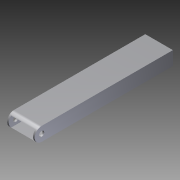
# Autodesk Inventor part: apendage arm
Saved by Autodesk Inventor 2012 (Build 160160000, 160)
## iProperties
Created: 2013-09-04
Part Number: apendage arm
Material: Default
Document SubType Name: Modeling
Designer: Bryce
Density: 1 g/cm^3
Author: Bryce
Autodesk Inventor part; units mm, degrees
ref_plane "YZ Plane" through (0, 0, 0) normal (1, 0, 0) x (0, 1, 0)
ref_plane "XZ Plane" through (0, 0, 0) normal (0, 1, 0) x (-1, 0, 0)
ref_plane "XY Plane" through (0, 0, 0) normal (0, 0, 1) x (1, 0, 0)
sketch "Sketch1" plane through (0, 0, 0) normal (0, 0, 1) x (1, 0, 0)
  line L0 (0, 0) -> (50.8, 0)
  line L1 (50.8, 0) -> (50.8, 25.4)
  line L2 (50.8, 25.4) -> (0, 25.4)
  line L3 (0, 25.4) -> (0, 0)
  line L4 (3.175, 3.175) -> (47.625, 3.175)
  line L5 (47.625, 3.175) -> (47.625, 22.225)
  line L6 (47.625, 22.225) -> (3.175, 22.225)
  line L7 (3.175, 22.225) -> (3.175, 3.175)
  dimension "d0" = 25.4
  dimension "d1" = 50.8
  dimension "d2" = 3.175
  dimension "d3" = 3.175
  dimension "d4" = 3.175
  dimension "d5" = 3.175
  constraints: 16 end point, 4 parallel, 2 horizontal, 2 perpendicular
  measures "d0" distance of L2.end L0.start
  measures "d1" distance of L0.start L0.end
  measures "d2" distance between parallel lines of L7 L3
  measures "d3" distance between parallel lines of L0 L4
  measures "d4" distance between parallel lines of L1 L5
  measures "d5" distance between parallel lines of L2 L6
extrude "Extrusion1" add sketch "Sketch1" along normal blind 254
sketch "Sketch2" plane through (50.8, 0, 0) normal (1, 0, 0) x (0, 0, -1)
  line L0 (-254, 25.4) -> (-254, 0) projected
  line L1 (0, 0) -> (-254, 0) projected
  line L2 (0, 0) -> (0, 25.4) projected
  line L3 (0, 25.4) -> (-254, 25.4) projected
  circle A0 centre (-241.3, 12.7) radius 4.7625
  arc A1 (-241.3, 25.4) -> (-241.3, 0) centre (-241.3, 12.7) ccw
  dimension "d8" = 9.525
  dimension "d9" = 12.7
  constraints: 2 centre point, 2 point on circle, 2 point on line, 2 tangent, 1 coincident
  measures "d8" diameter of A0
  measures "d9" distance from line of L0 A0.centre
extrude "Extrusion2" cut sketch "Sketch2" against normal blind 254 contours L3 A1 L0 | A1 L1 L0 | A0
equation "\"d2\" = d5"
equation "\"d3\" = d2"
equation "\"d4\" = d3"
body "Solid1"
